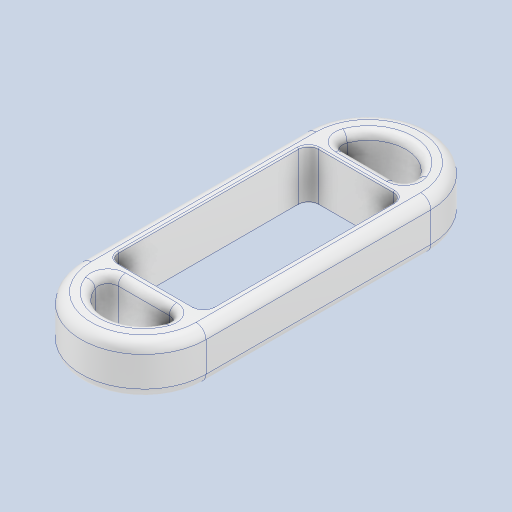
# Autodesk Inventor part: mod1
Saved by Autodesk Inventor 2024 (Build 280153000, 153)
## iProperties
Created: 2025-12-02
Part Number: mod1
Material: Aluminio 6061
Document SubType Name: Modeling
Designer: ANDRES
Density: 2.7 g/cm^3
Appearance: Aluminio - Plano
Author: ANDRES
## iProperties of the stored document mod1_3DPrint.ipt
Created: 2025-12-04
Part Number: mod1_3DPrint
Material: Genérico
Document SubType Name: Modeling
Designer: ANDRES
Density: 1 g/cm^3
Appearance: Valor por defecto
Author: ANDRES
Autodesk Inventor part; units mm, degrees
ref_plane "YZ Plane" through (0, 0, 0) normal (1, 0, 0) x (0, 1, 0)
ref_plane "XZ Plane" through (0, 0, 0) normal (0, 1, 0) x (-1, 0, 0)
ref_plane "XY Plane" through (0, 0, 0) normal (0, 0, 1) x (1, 0, 0)
sketch "Boceto1" plane through (0, 0, 0) normal (0, 1, 0) x (-1, 0, 0)
  line L0 (0, 45) -> (0, -45) construction
  line L1 (25, 45) -> (25, -45)
  line L2 (-25, -45) -> (-25, 45)
  arc A0 (25, 45) -> (-25, 45) centre (0, 45) ccw
  arc A1 (-25, -45) -> (25, -45) centre (0, -45) ccw
  circle A2 centre (0, -45) radius 15
  circle A3 centre (0, 45) radius 15
  line L3 (15, -45) -> (-15, -45)
  line L4 (94.5074, 0) -> (-76.0102, 0) construction
  line L5 (15, 45) -> (-15, 45)
  line L6 (-19, 40) -> (19, 40)
  line L7 (19, 40) -> (19, -40)
  line L8 (19, -40) -> (-19, -40)
  line L9 (-19, -40) -> (-19, 40)
  line L10 (-19, 40) -> (19, -40) construction
  line L11 (19, 40) -> (-19, -40) construction
  point P0 (0, 0)
  point P1 (0, 70)
  point P2 (0, -70)
  point P3 (0, -35)
  point P4 (-15, 45)
  point P5 (15, 45)
  dimension "largo" = 140
  dimension "d1" = 50
  dimension "espesor_junta" = 10
  dimension "d3" = 10
  dimension "d11" = 80
  dimension "d12" = 38
  dimension "d18" = 6
  constraints: 26 end point, 8 point on circle, 4 centre point, 4 horizontal, 4 midpoint, 4 tangent, 3 parallel, 2 concentric, 2 symmetric about line, 1 perpendicular, 1 vertical, 1 vertical alignment
  measures "largo" distance of point (0, 70) point (0, -70)
  measures "d1" distance between parallel lines of L2 L1
  measures "espesor_junta" radial gap between concentric circles of A1 A2
  measures "d3" radial gap between concentric circles of A0 A3
  measures "d11" distance of L6.end L7.end
  measures "d12" distance of L7.end L8.end
  measures "d18" distance between parallel lines of L7 L1
extrude "Extrusión2" add sketch "Boceto1" along normal blind 20 contours L1 A1 L2 A0 | A2 L8 L3 | A3 L5 L6
fillet "Empalme2" radius 4 8 edges at (0, 20, 70) (25, 20, 0) (0, 20, -70) (-25, 20, 0) (0, 0, 70) (25, 0, 0) (0, 0, -70) (-25, 0, 0)
fillet "Empalme3" radius 4 8 edges at (-19, 10, 40) (-19, 10, -40) (19, 10, -40) (19, 10, 40) (-15, 10, 45) (15, 10, 45) (-15, 10, -45) (15, 10, -45)
fillet "Empalme4" radius 3 16 edges at (13.5498, 20, -46.7437) (0, 20, -45) (-13.5498, 20, -46.7437) (0, 20, -60) (13.5498, 20, 46.7437) (0, 20, 60) (-13.5498, 20, 46.7437) (0, 20, 45) (13.5498, 0, -46.7437) (0, 0, -45) (-13.5498, 0, -46.7437) (0, 0, -60) (0, 0, 60) (-13.5498, 0, 46.7437) (0, 0, 45) (13.5498, 0, 46.7437)
fillet "Empalme5" radius 0.5 16 edges at (-17.8284, 20, -38.8284) (0, 20, -40) (17.8284, 20, -38.8284) (19, 20, 0) (17.8284, 20, 38.8284) (0, 20, 40) (-17.8284, 20, 38.8284) (-19, 20, 0) (-17.8284, 0, -38.8284) (0, 0, -40) (17.8284, 0, -38.8284) (19, 0, 0) (17.8284, 0, 38.8284) (0, 0, 40) (-17.8284, 0, 38.8284) (-19, 0, 0)
equation "\"d3\" = espesor_junta"
